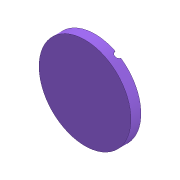
# Autodesk Inventor part: 50_ETL_Membrane_Mould_Upper_v0
Saved by Autodesk Inventor 2022 (Build 260153000, 153)
## iProperties
Created: 2021-12-31
Part Number: 50_ETL_Membrane_Mould_Upper_v0
Material: Generisch
Document SubType Name: Modeling
Designer: diederichbenedict
Density: 1 g/cm^3
Appearance: Violett
Author: diederichbenedict
Autodesk Inventor part; units mm, degrees
ref_plane "YZ Plane" through (0, 0, 0) normal (1, 0, 0) x (0, 1, 0)
ref_plane "XZ Plane" through (0, 0, 0) normal (0, 1, 0) x (-1, 0, 0)
ref_plane "XY Plane" through (0, 0, 0) normal (0, 0, 1) x (1, 0, 0)
sketch "Skizze1" plane through (0, 0, 0) normal (1, 0, 0) x (0, 1, 0)
  line L0 (4.655, 0) -> (-29.655, 0)
  line L1 (5, -1.0263) -> (5, 0)
  line L2 (-3.9492, 2.2) -> (-21.0508, 2.2)
  line L3 (-6.3, 0.7) -> (-18.7, 0.7)
  line L4 (-12.5, 1.3) -> (-12.5, 3.3)
  line L5 (4.655, 0) -> (-1, 0)
  line L6 (-18.5, 0.7) -> (-6.5, 0.7) construction
  line L7 (-6.5, 0.9) -> (-18.5, 0.9) construction
  line L8 (-18.5, 0.9) -> (-18.5, 0.7) construction
  line L9 (-18.5, 0.7) -> (-6.5, 0.9) construction
  line L10 (-6.5, 0.7) -> (-18.5, 0.9) construction
  line L11 (-6.3, 0.7) -> (-7.4658, 0.7) construction
  line L12 (-6.3, 0.7) -> (-6.4, 0.7)
  line L13 (-12.5, 1.3) -> (-12.5, 3.3)
  line L14 (-12.5, 3.3) -> (4.655, 3.3)
  line L15 (4.655, 3.3) -> (4.655, 0)
  line L16 (-3.9492, 2.2) -> (-21.0508, 2.2)
  line L17 (-5.7431, 0.4) -> (-4.5431, 1.6) construction
  line L18 (-4.1977, 1.6) -> (-20.8023, 1.6) construction
  line L19 (-4.1977, 1.6) -> (-3.1977, 0.6) construction
  line L20 (-4.1977, 1.6) -> (-20.8023, 1.6) construction
  line L21 (4.655, 3.3) -> (7.3306, 3.3)
  line L22 (7.3306, 3.3) -> (7.3306, -1.0263)
  line L23 (7.3306, -1.0263) -> (5.308, -1.0263)
  line L24 (4.655, 0) -> (4.705, 0)
  line L25 (4.705, 0) -> (5.3133, -1.0263)
  line L26 (-1, 0) -> (-3.6, 2.6)
  line L27 (-4.6, 2.6) -> (-5.9, 1.3)
  line L28 (-6.1, 1.1) -> (-18.9, 1.1)
  line L29 (-5.9, 1.3) -> (-12.5, 1.3)
  line L30 (-4.6, 2.6) -> (-3.6, 2.6)
  point P0 (0, 0)
  point P1 (5, -1.0263)
  point P2 (-2.1515, 0)
  point P3 (-5.8, 2.2)
  point P4 (-6.4, 0.9)
  point P5 (-4.8, 2.2)
  point P6 (-1.7515, 0)
  point P7 (-12.5, 2.2)
  point P8 (-5, 2.2)
  point P9 (-12.5, 2.2)
revolve "Umdrehung1" add sketch "Skizze1" angle 360 about axis through (0, -12.5, 1.3) along (0, 0, 1)
sketch "Skizze2" plane through (0, 0, 0) normal (1, 0, 0) x (0, 1, 0)
  line L0 (-30.3133, -1.0263) -> (5.3133, -1.0263) projected
  line L1 (-24, 0) -> (-1, 0) projected
  circle A0 centre (-12.5, -1.0263) radius 1.0263
  circle A1 centre (-12.5, -1.0263) radius 1.3923
  point P0 (0, 0)
  constraints: 2 centre point, 1 midpoint, 1 tangent
extrude "Extrusion1" cut sketch "Skizze2" against normal through all
pattern_circular "Runde Anordnung1" count 3 over 360 about axis through (0, -12.5, -0.5131) along (0, 0, -1) of "Extrusion1"
